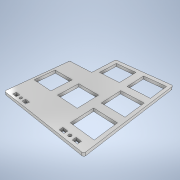
# Autodesk Inventor part: tc_base_plate
Saved by Autodesk Inventor 2020 (Build 240168000, 168)
## iProperties
Created: 2019-07-03
Part Number: tc_base_plate
Material: Acier, galvanisé
Document SubType Name: Modeling
Designer: Thibault
Density: 7.85 g/cm^3
Appearance: Aluminium - Poli
Author: Thibault
Autodesk Inventor part; units mm, degrees
ref_plane "YZ Plane" through (0, 0, 0) normal (1, 0, 0) x (0, 1, 0)
ref_plane "XZ Plane" through (0, 0, 0) normal (0, 1, 0) x (-1, 0, 0)
ref_plane "XY Plane" through (0, 0, 0) normal (0, 0, 1) x (1, 0, 0)
sketch "screw_anchor" plane through (0, 0, 0) normal (0, 0, 1) x (1, 0, 0)
  point P0 (61.1245, 15.5217)
  dimension "d155" = 14
  dimension "d156" = 19.05
  dimension "d157" = 19.05
  dimension "d158" = 19.05
  dimension "d159" = 28.575
  dimension "d160" = 19.05
  dimension "d161" = 2
  dimension "d162" = 2
  dimension "d163" = 2
  dimension "d164" = 2
  dimension "d165" = 2
  dimension "d166" = 1
  dimension "d167" = 5
  dimension "d168" = 5
  dimension "d169" = 4
  dimension "d258" = 5.05
  dimension "d259" = 5.05
sketch "anchor" plane through (0, 0, 0) normal (0, 0, 1) x (1, 0, 0)
  circle A0 centre (94.2814, 48.5827) radius 0.85
  line L0 (91.2814, 49.5827) -> (87.2814, 49.5827)
  line L1 (87.2814, 49.5827) -> (87.2814, 47.5827)
  line L2 (87.2814, 47.5827) -> (91.2814, 47.5827)
  line L3 (91.2814, 47.5827) -> (91.2814, 49.5827)
  line L4 (101.2814, 49.5827) -> (97.2814, 49.5827)
  line L5 (97.2814, 49.5827) -> (97.2814, 47.5827)
  line L6 (97.2814, 47.5827) -> (101.2814, 47.5827)
  line L7 (101.2814, 47.5827) -> (101.2814, 49.5827)
  line L8 (91.2814, 49.5827) -> (97.2814, 47.5827) construction
  line L9 (97.2814, 49.5827) -> (91.2814, 47.5827) construction
  line L10 (87.2814, 51.1827) -> (101.2814, 51.1827)
  point P0 (103.5798, 50.1132)
  point P1 (94.2814, 48.5827)
  dimension "d258" = 5.05
  dimension "d259" = 5.05
  dimension "d226" = 1.7
  dimension "d230" = 4
  dimension "d231" = 2
  dimension "d237" = 4
  dimension "d245" = 1.6
  dimension "d247" = 6
  measures "d226" diameter of A0
  measures "d230" distance of L2.end L1.end
  measures "d231" distance of L1.end L0.end
  measures "d237" distance of L6.end L5.end
  measures "d245" distance between parallel lines of L0 L10
  measures "d247" distance between parallel lines of L5 L3
sketch "Anchor (screw side)" plane through (0, 0, 0) normal (0, 0, 1) x (1, 0, 0)
  circle A0 centre (93.7814, 50.2592) radius 0.85
  line L0 (91.2814, 51.2592) -> (88.2814, 51.2592)
  line L1 (88.2814, 51.2592) -> (88.2814, 49.2592)
  line L2 (88.2814, 49.2592) -> (91.2814, 49.2592)
  line L3 (91.2814, 49.2592) -> (91.2814, 51.2592)
  line L4 (99.2814, 51.2592) -> (96.2814, 51.2592)
  line L5 (96.2814, 51.2592) -> (96.2814, 49.2592)
  line L6 (96.2814, 49.2592) -> (99.2814, 49.2592)
  line L7 (99.2814, 49.2592) -> (99.2814, 51.2592)
  line L8 (91.2814, 51.2592) -> (96.2814, 49.2592) construction
  line L9 (96.2814, 51.2592) -> (91.2814, 49.2592) construction
  line L10 (86.6814, 52.8592) -> (100.8814, 52.8592) construction
  line L11 (100.8814, 52.8592) -> (100.8814, 47.6592) construction
  line L12 (100.8814, 47.6592) -> (86.6814, 47.6592) construction
  line L13 (86.6814, 47.6592) -> (86.6814, 52.8592) construction
  point P0 (103.5798, 50.1132)
  dimension "d27" = 1.7
  dimension "d28" = 3
  dimension "d29" = 2
  dimension "d30" = 3
  dimension "d32" = 5
  dimension "d34" = 1.6
  dimension "d35" = 1.6
  dimension "d36" = 1.6
  dimension "d37" = 1.6
  measures "d27" diameter of A0
  measures "d28" distance of L2.end L1.end
  measures "d29" distance of L1.end L0.end
  measures "d30" distance of L6.end L5.end
  measures "d32" distance between parallel lines of L5 L3
  measures "d34" distance between parallel lines of L0 L10
  measures "d35" distance between parallel lines of L12 L2
  measures "d36" distance between parallel lines of L11 L7
  measures "d37" distance between parallel lines of L13 L1
sketch "Anchor (nut side)" plane through (0, 0, 0) normal (0, 0, 1) x (1, 0, 0)
  line L0 (10, 0) -> (8.35, 0)
  line L1 (8.35, 0) -> (8.35, -2.5)
  line L2 (8.35, -2.5) -> (9.15, -2.5)
  line L3 (9.15, -2.5) -> (9.15, -4.5)
  line L4 (5.85, -4.5) -> (5.85, -2.5)
  line L5 (5.85, -2.5) -> (6.65, -2.5)
  line L6 (6.65, -2.5) -> (6.65, 0)
  line L7 (6.65, 0) -> (5, 0)
  line L8 (2, 0) -> (2, 1.75)
  line L9 (2, 0) -> (3, 0) construction
  line L10 (2.25, 2) -> (4.75, 2)
  line L11 (5, 1.75) -> (5, 0)
  line L12 (5, 2) -> (7, 2) construction
  line L13 (10, 0) -> (10, 1.75)
  line L14 (10.25, 2) -> (12.75, 2)
  line L15 (13, 1.75) -> (13, 0)
  line L16 (0, 0) -> (2, 0)
  line L17 (13, 0) -> (15, 0)
  line L18 (5.85, -4.5) -> (6.65, -4.5)
  line L19 (9.15, -4.5) -> (8.35, -4.5)
  line L20 (6.65, -4.5) -> (6.65, -6)
  line L21 (8.35, -4.5) -> (8.35, -6)
  arc A0 (2.25, 2) -> (2, 1.75) centre (2.25, 1.75) ccw
  arc A1 (5, 1.75) -> (4.75, 2) centre (4.75, 1.75) ccw
  arc A2 (10.25, 2) -> (10, 1.75) centre (10.25, 1.75) ccw
  arc A3 (13, 1.75) -> (12.75, 2) centre (12.75, 1.75) ccw
  line L22 (7.15, -6.5) -> (7.85, -6.5)
  arc A4 (6.65, -6) -> (7.15, -6.5) centre (7.15, -6) ccw
  arc A5 (7.85, -6.5) -> (8.35, -6) centre (7.85, -6) ccw
  point P0 (9.1321, -0.6227)
  point P1 (2, 2)
  point P2 (10, 2)
  point P3 (13, 2)
  point P4 (6.65, -6.5)
  point P5 (8.35, -6.5)
  dimension "d3" = 2
  dimension "d5" = 3
  dimension "d7" = 5
  dimension "d8" = 3
  dimension "d10" = 1.65
  dimension "d11" = 2.5
  dimension "d12" = 0.8
  dimension "d13" = 2
  dimension "d14" = 0.8
  dimension "d15" = 1.7
  dimension "d16" = 2.5
  dimension "d18" = 2
  dimension "d19" = 0.8
  dimension "d20" = 0.8
  dimension "d21" = 2
  dimension "d22" = 2
  dimension "d23" = 1.7
  dimension "d24" = 2
  dimension "d25" = 0.25
  dimension "d38" = 2
  dimension "d39" = 0.5
  measures "d3" distance of L16.start L8.start
  measures "d5" distance of point (2, 2) L12.start
  measures "d7" distance of L7.end L0.start
  measures "d8" distance of point (10, 2) point (13, 2)
  measures "d10" distance of L0.start L0.end
  measures "d11" distance of L0.end L1.end
  measures "d12" distance of L1.end L2.end
  measures "d13" distance of L2.end L3.end
  measures "d14" distance of L4.end L5.end
  measures "d15" distance of L6.end L0.end
  measures "d16" distance of L5.end L6.end
  measures "d18" distance of L15.end L17.end
  measures "d19" distance of L4.start L18.end
  measures "d20" distance of L3.end L19.end
  measures "d21" distance of L18.end point (6.65, -6.5)
  measures "d22" distance of L19.end point (8.35, -6.5)
  measures "d23" distance of L18.end L19.end
  measures "d24" distance of L4.start L4.end
  measures "d25" radius of A0
  measures "d38" distance between parallel lines of L16 L10
  measures "d39" radius of A4
sketch "Esquisse2" plane through (0, 0, 0) normal (0, 1, 0) x (-1, 0, 0)
  line L0 (17.2703, -7.6777) -> (3.2703, -7.6777)
  line L1 (3.2703, -7.6777) -> (3.2703, 6.3223)
  line L2 (3.2703, 6.3223) -> (17.2703, 6.3223)
  line L3 (17.2703, 6.3223) -> (17.2703, -7.6777)
  line L4 (17.2703, -45.7777) -> (3.2703, -45.7777)
  line L5 (3.2703, -45.7777) -> (3.2703, -31.7777)
  line L6 (3.2703, -31.7777) -> (17.2703, -31.7777)
  line L7 (17.2703, -31.7777) -> (17.2703, -45.7777)
  line L8 (17.2703, -26.7277) -> (3.2703, -26.7277)
  line L9 (3.2703, -26.7277) -> (3.2703, -12.7277)
  line L10 (3.2703, -12.7277) -> (17.2703, -12.7277)
  line L11 (17.2703, -12.7277) -> (17.2703, -26.7277)
  line L12 (36.3203, -45.7777) -> (22.3203, -45.7777)
  line L13 (22.3203, -45.7777) -> (22.3203, -31.7777)
  line L14 (22.3203, -31.7777) -> (36.3203, -31.7777)
  line L15 (36.3203, -31.7777) -> (36.3203, -45.7777)
  line L16 (36.3203, -16.2876) -> (22.3203, -16.2876)
  line L17 (22.3203, -16.2876) -> (22.3203, -2.2876)
  line L18 (22.3203, -2.2876) -> (36.3203, -2.2876)
  line L19 (36.3203, -2.2876) -> (36.3203, -16.2876)
  line L20 (55.3703, -16.2876) -> (41.3703, -16.2876)
  line L21 (41.3703, -16.2876) -> (41.3703, -2.2876)
  line L22 (41.3703, -2.2876) -> (55.3703, -2.2876)
  line L23 (55.3703, -2.2876) -> (55.3703, -16.2876)
  line L24 (56.3703, -28.7277) -> (40.3203, -28.7277)
  line L25 (39.3203, -29.7277) -> (39.3203, -47.7777)
  line L26 (38.3203, -48.7777) -> (2.2703, -48.7777)
  arc A0 (38.3203, -48.7777) -> (39.3203, -47.7777) centre (38.3203, -47.7777) ccw
  arc A1 (40.3203, -28.7277) -> (39.3203, -29.7277) centre (40.3203, -29.7277) ccw
  line L27 (1.2703, -47.7777) -> (1.2703, 12.9223)
  line L28 (57.3703, -27.7277) -> (57.3703, 12.9223)
  arc A2 (1.2703, -47.7777) -> (2.2703, -48.7777) centre (2.2703, -47.7777) ccw
  arc A3 (56.3703, -28.7277) -> (57.3703, -27.7277) centre (56.3703, -27.7277) ccw
  line L29 (56.3703, 13.9223) -> (2.2703, 13.9223)
  arc A4 (57.3703, 12.9223) -> (56.3703, 13.9223) centre (56.3703, 12.9223) ccw
  arc A5 (2.2703, 13.9223) -> (1.2703, 12.9223) centre (2.2703, 12.9223) ccw
  circle A6 centre (46.8203, 11.3223) radius 0.85
  line L30 (44.3203, 12.3223) -> (41.3203, 12.3223)
  line L31 (41.3203, 12.3223) -> (41.3203, 10.3223)
  line L32 (41.3203, 10.3223) -> (44.3203, 10.3223)
  line L33 (44.3203, 10.3223) -> (44.3203, 12.3223)
  line L34 (52.3203, 12.3223) -> (49.3203, 12.3223)
  line L35 (49.3203, 12.3223) -> (49.3203, 10.3223)
  line L36 (49.3203, 10.3223) -> (52.3203, 10.3223)
  line L37 (52.3203, 10.3223) -> (52.3203, 12.3223)
  line L38 (44.3203, 12.3223) -> (49.3203, 10.3223) construction
  line L39 (49.3203, 12.3223) -> (44.3203, 10.3223) construction
  line L40 (39.7203, 13.9223) -> (53.9203, 13.9223) construction
  line L41 (53.9203, 13.9223) -> (53.9203, 8.7223) construction
  line L42 (53.9203, 8.7223) -> (39.7203, 8.7223) construction
  line L43 (39.7203, 8.7223) -> (39.7203, 13.9223) construction
  circle A7 centre (11.8203, 11.3223) radius 0.85
  line L44 (9.3203, 12.3223) -> (6.3203, 12.3223)
  line L45 (6.3203, 12.3223) -> (6.3203, 10.3223)
  line L46 (6.3203, 10.3223) -> (9.3203, 10.3223)
  line L47 (9.3203, 10.3223) -> (9.3203, 12.3223)
  line L48 (17.3203, 12.3223) -> (14.3203, 12.3223)
  line L49 (14.3203, 12.3223) -> (14.3203, 10.3223)
  line L50 (14.3203, 10.3223) -> (17.3203, 10.3223)
  line L51 (17.3203, 10.3223) -> (17.3203, 12.3223)
  line L52 (9.3203, 12.3223) -> (14.3203, 10.3223) construction
  line L53 (14.3203, 12.3223) -> (9.3203, 10.3223) construction
  line L54 (4.7203, 13.9223) -> (18.9203, 13.9223) construction
  line L55 (18.9203, 13.9223) -> (18.9203, 8.7223) construction
  line L56 (18.9203, 8.7223) -> (4.7203, 8.7223) construction
  line L57 (4.7203, 8.7223) -> (4.7203, 13.9223) construction
  point P0 (39.3203, -28.7277)
  point P1 (39.3203, -48.7777)
  point P2 (12.982, -48.7777)
  point P3 (57.3703, -28.7277)
  point P4 (1.2703, -48.7777)
  point P5 (1.2703, 13.9223)
  dimension "d257" = 35
  dimension "d108" = 14
  dimension "d109" = 19.05
  dimension "d110" = 19.05
  dimension "d111" = 19.05
  dimension "d114" = 19.05
  dimension "d116" = 3
  dimension "d117" = 3
  dimension "d123" = 2
  dimension "d181" = 2
  dimension "d190" = 2
  dimension "d191" = 1
  dimension "d258" = 5.05
  dimension "d259" = 5.05
  dimension "d260" = 4
  dimension "d261" = 1
  constraints: 60 end point, 12 parallel, 12 point on circle, 12 tangent, 11 equal length, 11 point on line, 10 horizontal, 7 perpendicular, 6 centre point, 5 collinear, 2 vertical, 1 equal radius
  measures "d108" distance of L1.end L2.end
  measures "d109" distance of L8.end L4.end
  measures "d110" distance of L0.end L8.end
  measures "d111" distance of L4.start L12.start
  measures "d114" distance of L18.end L22.end
  measures "d116" distance between parallel lines of L26 L4
  measures "d117" distance between parallel lines of L25 L15
  measures "d123" distance between parallel lines of L8 L24
  measures "d181" distance between parallel lines of L27 L5
  measures "d190" distance between parallel lines of L28 L23
  measures "d191" radius of A2
  measures "d261" radius of A4
extrude "Base" add sketch "Esquisse2" along normal blind 2
ref_plane "Plan de construction4" through (-10.2703, 0, -45.7777) normal (-1, 0, 0) x (0, 0, 1)
ref_plane "Plan de construction5" through (-29.3203, 0, -31.7777) normal (1, 0, 0) x (0, 0, -1)
ref_plane "Plan de construction6" through (-48.3703, 0, -16.2876) normal (-1, 0, 0) x (0, 0, 1)
derived "shared_parameters.ipt"
